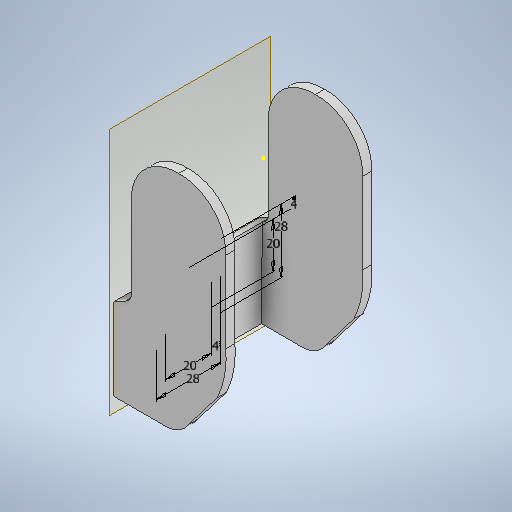
# Autodesk Inventor part: horn-connector-2
Saved by Autodesk Inventor 2025 (Build 290162000, 162)
## iProperties
Created: 2024-05-27
Part Number: horn-connector-2
Material: Generic
Document SubType Name: Modeling
Designer: hifzh
Density: 1 g/cm^3
Appearance: Default
Author: hifzh
Autodesk Inventor part; units mm, degrees
ref_plane "XZ Plane" through (0, 0, 0) normal (0, 1, 0) x (-1, 0, 0)
sketch "Sketch1" plane through (0, 0, 0) normal (0, 0, 1) x (1, 0, 0)
  arc A0 (0, 39.704) -> (-20.705, 19) centre (-0.7179, 19.7169) ccw
  arc A1 (20.705, 19) -> (0, 39.704) centre (0.7179, 19.7169) ccw
  arc A2 (-23.3216, -20.418) -> (-20.705, -15.169) centre (-25.1908, -16.2095) ccw
  line L0 (-28.3702, -23.154) -> (-23.3216, -20.418)
  line L1 (-20.705, -15.169) -> (-20.705, 19)
  line L2 (20.705, -16.549) -> (20.705, 19)
  line L3 (-28.3702, -23.154) -> (-28.3702, -59.154)
  arc A3 (16.8635, -37.0914) -> (20.705, -16.549) centre (-19.3207, -19.6945) ccw
  arc A4 (-5.6175, -59.154) -> (4.2559, -53.5861) centre (-5.6175, -47.6161) ccw
  line L4 (16.8635, -37.0914) -> (4.2559, -53.5861)
  line L5 (-5.6175, -59.154) -> (-28.3702, -59.154)
  point P0 (0, 0)
  point P1 (0, 19)
  point P2 (4.2559, -53.5861)
  dimension "d1" = 20
  dimension "d2" = 20
  dimension "d9" = 36
  constraints: 12 end point, 10 point on circle, 5 centre point, 3 vertical, 1 horizontal
  measures "d1" radius of A0
  measures "d2" radius of A1
  measures "d9" distance of L0.start L3.end
extrude "Extrusion1" add sketch "Sketch1" along normal blind 64
ref_plane "Work Plane2" through (0, 0, 32) normal (0, 0, 1) x (1, 0, 0)
sketch "Sketch5" plane through (0, 0, 32) normal (0, 0, 1) x (1, 0, 0)
  arc A0 (0, 39.704) -> (-20.705, 19) centre (-0.7179, 19.7169) ccw
  arc A1 (20.705, 19) -> (0, 39.704) centre (0.7179, 19.7169) ccw
  line L0 (-20.705, -15.169) -> (-20.705, 19)
  line L1 (20.705, -16.549) -> (20.705, 19)
  arc A2 (16.8635, -37.0914) -> (20.705, -16.549) centre (-19.3207, -19.6945) ccw
  arc A3 (-5.6175, -59.154) -> (4.2559, -53.5861) centre (-5.6175, -47.6161) ccw
  line L2 (16.8635, -37.0914) -> (4.2559, -53.5861)
  arc A4 (-23.3216, -20.418) -> (-20.705, -15.169) centre (-25.1908, -16.2095) ccw projected
  line L3 (-5.6175, -59.154) -> (-23.6175, -59.154)
  line L4 (-28.3702, -59.154) -> (-5.6175, -59.154) projected
  line L5 (-23.6175, -59.154) -> (-23.3216, -20.418)
  line L6 (-23.3216, -20.418) -> (-28.3702, -23.154) projected
  arc A5 (-23.3216, -20.418) -> (-20.705, -15.169) centre (-25.1908, -16.2095) ccw
  point P0 (0, 0)
  point P1 (0, 0)
  point P2 (0, 19)
  point P3 (6.3637, -44.409)
  point P4 (4.2559, -53.5861)
  dimension "d14" = 20
  dimension "d15" = 20
  dimension "d19" = 18
  constraints: 10 end point, 10 point on circle, 5 centre point, 2 point on line, 2 vertical, 1 concentric
  measures "d14" radius of A0
  measures "d15" radius of A1
  measures "d19" distance of L3.start L3.end
extrude "Extrusion2" cut sketch "Sketch5" along normal mid plane 56
ref_plane "Work Plane4" through (-26.9875, 0, 0) normal (1, 0, 0) x (0, 1, 0)
sketch "Sketch6" plane through (-26.9875, 0, 0) normal (1, 0, 0) x (0, 1, 0)
  line L0 (-21.3394, 46.6838) -> (-49.3394, 46.6838)
  line L1 (-49.3394, 46.6838) -> (-49.3394, 18.6838)
  line L2 (-49.3394, 18.6838) -> (-21.3394, 18.6838)
  line L3 (-21.3394, 18.6838) -> (-21.3394, 46.6838)
  line L4 (-25.3394, 42.6838) -> (-45.3394, 42.6838)
  line L5 (-45.3394, 42.6838) -> (-45.3394, 22.6838)
  line L6 (-45.3394, 22.6838) -> (-25.3394, 22.6838)
  line L7 (-25.3394, 22.6838) -> (-25.3394, 42.6838)
  point P0 (0, 0)
  point P1 (-25.3394, 32.6838)
  point P2 (-35.3394, 18.6838)
  point P3 (-35.3394, 22.6838)
  dimension "d24" = 20
  dimension "d25" = 28
  dimension "d26" = 20
  dimension "d27" = 28
  dimension "d28" = 4
  dimension "d29" = 4
  constraints: 16 end point, 4 parallel, 3 midpoint, 2 horizontal, 2 perpendicular
  measures "d24" distance of L4.end L5.end
  measures "d25" distance of L0.end L1.end
  measures "d26" distance of L5.end L6.end
  measures "d27" distance of L1.end L2.end
  measures "d28" distance from line of L3 point (-25.339, 32.684)
  measures "d29" distance of point (-35.339, 18.684) point (-35.339, 22.684)
body "Solid1"
